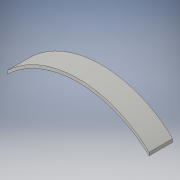
# Autodesk Inventor part: ClampLip
Saved by Autodesk Inventor 2016 (Build 200138000, 138)
## iProperties
Created: 2016-08-29
Part Number: ClampLip
Material: Generic
Document SubType Name: Modeling
Designer: yash
Density: 1 g/cm^3
Appearance: Default
Author: yash
Autodesk Inventor part; units mm, degrees
ref_plane "YZ Plane" through (0, 0, 0) normal (1, 0, 0) x (0, 1, 0)
ref_plane "XZ Plane" through (0, 0, 0) normal (0, 1, 0) x (-1, 0, 0)
ref_plane "XY Plane" through (0, 0, 0) normal (0, 0, 1) x (1, 0, 0)
sketch "Sketch1" plane through (0, 0, 0) normal (0, 0, 1) x (1, 0, 0)
  line L0 (0, 0) -> (76.2, 0) construction
  line L1 (0, 0) -> (76.2, 0) construction
  line L2 (0, 0) -> (38.1, 0) construction
  line L3 (38.1, 0) -> (38.1, 15.24) construction
  line L4 (38.1, 15.24) -> (38.1, 16.9672) construction
  arc A0 (76.2, 0) -> (0, 0) centre (38.1, -40.005) ccw
  line L5 (0, 0) -> (0, 1.7272) construction
  line L6 (76.2, 0) -> (76.2, 1.7272) construction
  arc A1 (76.2, 1.7272) -> (0, 1.7272) centre (38.1, -38.2778) ccw
  line L7 (0, 1.7272) -> (0, 0)
  line L8 (76.2, 1.7272) -> (76.2, 0)
  dimension "d0" = 76.2
  dimension "d1" = 0
  dimension "d2" = 38.1
  dimension "d3" = 15.24
  dimension "d4" = 1.7272
  dimension "d5" = 1.7272
  dimension "d6" = 1.7272
  constraints: 18 end point, 6 point on circle, 4 vertical, 2 centre point, 2 collinear, 2 horizontal, 1 coincident, 1 midpoint, 1 perpendicular, 1 point on line
  measures "d0" distance of L0.start L0.end
  measures "d1" distance between parallel lines of L0 L1
  measures "d2" distance of L2.start L2.end
  measures "d3" distance of L2.end L3.end
  measures "d4" distance of L3.end L4.end
  measures "d5" distance of L2.start L5.end
  measures "d6" distance of L1.end L6.end
extrude "Extrusion1" add sketch "Sketch1" along normal blind 12.7
equation "\"d2\" = 0.5 * d0"
equation "\"d3\" = 0.2 * d0"
body "Solid1"
